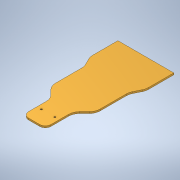
# Autodesk Inventor part: base_plate
Saved by Autodesk Inventor 2020 (Build 240168000, 168)
## iProperties
Created: 2020-03-15
Part Number: base_plate
Material: Acrylic, Clear
Document SubType Name: Modeling
Designer: 0x6f736f646f
Density: 1.19 g/cm^3
Appearance: Brass - Satin
Author: 0x6f736f646f
Autodesk Inventor part; units mm, degrees
ref_plane "YZ Plane" through (0, 0, 0) normal (1, 0, 0) x (0, 1, 0)
ref_plane "XZ Plane" through (0, 0, 0) normal (0, 1, 0) x (-1, 0, 0)
sketch "Sketch1" plane through (0, 0, 0) normal (0, 1, 0) x (-1, 0, 0)
  line L0 (0, -154.7214) -> (0, -200)
  line L1 (0, -200) -> (-100, -200)
  line L2 (-100, -200) -> (-100, -154.7214)
  line L3 (-60, 0) -> (-40, 0)
  line L4 (-2.1115, -145.7771) -> (-7.8885, -134.2229)
  line L5 (-10, -125.2786) -> (-10, -78.2843)
  line L6 (-15.8579, -64.1421) -> (-24.1421, -55.8579)
  line L7 (-30, -41.7157) -> (-30, -10)
  line L8 (-70, -10) -> (-70, -41.7157)
  line L9 (-75.8579, -55.8579) -> (-84.1421, -64.1421)
  line L10 (-90, -78.2843) -> (-90, -125.2786)
  line L11 (-92.1115, -134.2229) -> (-97.8885, -145.7771)
  arc A0 (-30, -41.7157) -> (-24.1421, -55.8579) centre (-10, -41.7157) ccw
  arc A1 (-75.8579, -55.8579) -> (-70, -41.7157) centre (-90, -41.7157) ccw
  arc A2 (-84.1421, -64.1421) -> (-90, -78.2843) centre (-70, -78.2843) ccw
  arc A3 (-10, -78.2843) -> (-15.8579, -64.1421) centre (-30, -78.2843) ccw
  arc A4 (-10, -125.2786) -> (-7.8885, -134.2229) centre (10, -125.2786) ccw
  arc A5 (-92.1115, -134.2229) -> (-90, -125.2786) centre (-110, -125.2786) ccw
  arc A6 (-97.8885, -145.7771) -> (-100, -154.7214) centre (-80, -154.7214) ccw
  arc A7 (0, -154.7214) -> (-2.1115, -145.7771) centre (-20, -154.7214) ccw
  arc A8 (-30, -10) -> (-40, 0) centre (-40, -10) ccw
  arc A9 (-60, 0) -> (-70, -10) centre (-60, -10) ccw
  point P0 (0, 0)
  point P1 (-100, 0)
  point P2 (0, -150)
  point P3 (-10, -130)
  point P4 (-10, -70)
  point P5 (-30, -50)
  point P6 (-30, 0)
  point P7 (-70, 0)
  point P8 (-70, -50)
  point P9 (-90, -70)
  point P10 (-90, -130)
  point P11 (-100, -150)
  point P12 (0, 0)
  dimension "d23" = 50
  dimension "d24" = 60
  dimension "d25" = 60
  dimension "d26" = 50
  dimension "d27" = 50
  dimension "d28" = 50
  dimension "d29" = 20
  dimension "d30" = 20
  dimension "d31" = 40
  dimension "d32" = 100
  dimension "d34" = 10
  dimension "d35" = 10
  dimension "d36" = 20
  dimension "d37" = 200
  dimension "d38" = 20
  dimension "d39" = 10
  constraints: 24 end point, 24 point on line, 20 point on circle, 20 tangent, 10 centre point, 8 equal radius, 4 perpendicular, 3 vertical, 1 coincident, 1 parallel
  measures "d23" distance of point (-30, -50) point (-30, 0)
  measures "d24" distance of point (-10, -130) point (-10, -70)
  measures "d25" distance of point (-90, -70) point (-90, -130)
  measures "d26" distance of point (-70, 0) point (-70, -50)
  measures "d27" distance of L1.end point (-100, -150)
  measures "d28" distance of L0.end point (0, -150)
  measures "d29" vertical distance of point (-10, -130) point (0, -150)
  measures "d30" vertical distance of point (-100, -150) point (-90, -130)
  measures "d31" distance between parallel lines of L8 L7
  measures "d32" distance between parallel lines of L2 L0
  measures "d34" distance between parallel lines of L0 L5
  measures "d35" distance between parallel lines of L2 L10
  measures "d36" distance between parallel lines of L5 L7
  measures "d37" distance between parallel lines of L1 L3
  measures "d38" radius of A0
  measures "d39" radius of A8
extrude "Extrusion2" add sketch "Sketch1" against normal blind 3
ref_plane "Work Plane1" through (0, 0, -25) normal (0, 0, 1) x (1, 0, 0)
sketch "Sketch8" plane through (0, 0, 0) normal (0, 1, 0) x (1, 0, 0)
  line L0 (70, 10) -> (70, 41.7157) projected
  line L1 (30, 41.7157) -> (30, 10) projected
  line L2 (40, 0) -> (60, 0) projected
  point P0 (0, 0)
  point P1 (38, 25)
  point P2 (62, 25)
  dimension "d117" = 8
  dimension "d118" = 8
  dimension "d119" = 25
  dimension "d120" = 25
  measures "d117" distance from line of L0 point (62, 25)
  measures "d118" distance from line of L1 point (38, 25)
  measures "d119" distance from line of L2 point (38, 25)
  measures "d120" distance from line of L2 point (62, 25)
hole "Hole2" at (38, 0, -25) at (62, 0, -25) direction (0, -1, 0) diameter 3 end through all
thread "Thread1" size "M3x0.5" class "6H" standard "ANSI Metric M Profile" length 3
thread "Thread2" size "M3x0.5" class "6H" standard "ANSI Metric M Profile" full length
body "Solid2"
